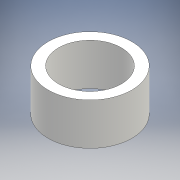
# Autodesk Inventor part: ドライメットブッシュ 内径6長さ4
Saved by Autodesk Inventor 2016 (Build 200138000, 138)
## iProperties
Created: 2019-11-12
Part Number: ドライメットブッシュ 内径6長さ4
Material: 一般
Document SubType Name: Modeling
Designer: mozar
Density: 1 g/cm^3
Appearance: 既定
Author: mozar
Autodesk Inventor part; units mm, degrees
ref_plane "YZ Plane" through (0, 0, 0) normal (1, 0, 0) x (0, 1, 0)
ref_plane "XZ Plane" through (0, 0, 0) normal (0, 1, 0) x (-1, 0, 0)
ref_plane "XY Plane" through (0, 0, 0) normal (0, 0, 1) x (1, 0, 0)
sketch "スケッチ1" plane through (0, 0, 0) normal (0, 0, 1) x (1, 0, 0)
  circle A0 centre (0, 0) radius 3
  circle A1 centre (0, 0) radius 4
  dimension "d0" = 6
  dimension "d1" = 8
  constraints: 2 centre point, 2 coincident
  measures "d0" diameter of A0
  measures "d1" diameter of A1
extrude "押し出し1" add sketch "スケッチ1" against normal blind 4
